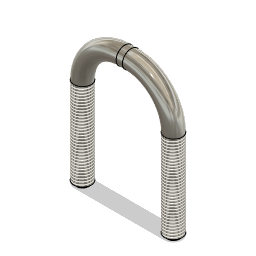
0.880.0738 - Etrier de 10x50x65 - IGTE 21400_17 Rep. 64 (Autodesk Fusion 360 design; units mm, degrees)
Autodesk Fusion 360 part; units mm, degrees
note: some values were not read from the file. Chosen so that the rebuilt part matches the saved one: which face or edge a step refers to; how an offset face is resized.
sketch "Sketch1" plane through (0, 0, 0) normal (0, 0, 1) x (1, 0, 0)
  circle A0 centre (0, 0) radius 19 construction
  circle A1 centre (0, 0) radius 24 construction
  line L0 (-24, 0.0214) -> (24, 0.0214) construction
  line L1 (0, 0) -> (0, -50) construction
  line L2 (-25.5, 0) -> (-25.5, -50)
  line L3 (25.5, 0) -> (25.5, -50)
  line L4 (0, 0) -> (0, 24) construction
  line L5 (-25.5, 0) -> (-25.5, 0.25)
  line L6 (0, 24) -> (-1.75, 24)
  arc A2 (-1.75, 24) -> (-25.5, 0.25) centre (-1.75, 0.25) ccw
  arc A3 (25.5, 0.25) -> (1.75, 24) centre (1.75, 0.25) ccw
  line L7 (0, 24) -> (1.75, 24)
  line L8 (25.5, 0) -> (25.5, 0.25)
  dimension "d1" = 38
  dimension "d2" = 5
  dimension "d3" = 50
  dimension "d4" = 25.5
  dimension "d5" = 25.5
  dimension "d6" = 23.75
  constraint coincident A0.centre A1.centre
  constraint coincident A1 L0.start
  constraint coincident A1 L0.end
  constraint horizontal L0
  constraint coincident A1 L4.end
  constraint perpendicular L0 L4
  constraint parallel L2 L5
  constraint tangent A1 L6
  constraint perpendicular L5 L6
  constraint tangent L6 A2
  constraint tangent L5 A2
  constraint symmetric L4 L6.end A3.end
  constraint symmetric L4 L5.end A3.start
  constraint symmetric L4 A2 A3
  constraint tangent A3 L8
  measures "d1" diameter of A0
  measures "d3" distance of A0.centre L1.end
  measures "d6" radius of A2
sketch "Sketch2" plane through (0, 0, 0) normal (1, 0, 0) x (0, 0, -1)
  circle A0 centre (0, 24) radius 5
  point P0 (0, 24)
  dimension "d7" = 10
  constraint coincident P0 A0.centre
  measures "d7" diameter of A0
sweep "Sweep1" add profiles "Sketch2" path "Sketch1" along L3 L8 A3 L7 L6 A2 L5 L2 section 1
chamfer "Chamfer1" distance 1.5 angle 45 2 edges at (-27.3081, -50, 4.6616) (23.6919, -50, 4.6616)
thread "Thread1" "ISO Metric profile 10.0 M10x1.5 6g" major diameter 9.85 minor diameter 8.141 pitch 1.5 angle 60 resizes the face on face at (-25.0022, -32.25, -4.9752)
thread "Thread2" "ISO Metric profile 10.0 M10x1.5 6g"
